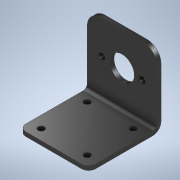
# Autodesk Inventor part: Pad dong co 775
Saved by Autodesk Inventor 2020 (Build 240168000, 168)
## iProperties
Created: 2021-05-25
Part Number: Pad dong co 775
Material: Generic
Document SubType Name: Sheet Metal
Designer: admin
Density: 1 g/cm^3
Sheet Metal Rule: Default_mm
Appearance: Glossy - Black
Author: admin
Autodesk Inventor part; units mm, degrees
ref_plane "YZ Plane" through (0, 0, 0) normal (1, 0, 0) x (0, 1, 0)
ref_plane "XZ Plane" through (0, 0, 0) normal (0, 1, 0) x (-1, 0, 0)
ref_plane "XY Plane" through (0, 0, 0) normal (0, 0, 1) x (1, 0, 0)
sketch "Sketch1" plane through (0, 0, 0) normal (0, 0, 1) x (1, 0, 0)
  line L0 (-25, -26) -> (25, -26)
  line L1 (25, -26) -> (25, 26)
  line L2 (25, 26) -> (-25, 26)
  line L3 (-25, 26) -> (-25, -26)
  line L4 (-25, -26) -> (25, 26) construction
  line L5 (25, -26) -> (-25, 26) construction
  circle A0 centre (0, 2) radius 8.8
  circle A1 centre (-14.5, 2) radius 2.25
  circle A2 centre (14.5, 2) radius 2.25
  point P0 (0, 0)
  dimension "d0" = 50
  dimension "d1" = 52
  dimension "d2" = 17.6
  dimension "d3" = 24
  dimension "d4" = 4.5
  dimension "d5" = 4.5
  dimension "d6" = 29
  dimension "d7" = 14.5
  dimension "d8" = 24
  dimension "d9" = 24
  dimension "d10" = 25
  measures "d0" distance of L2.end L1.end
  measures "d1" distance of L1.end L0.end
  measures "d2" diameter of A0
  measures "d3" distance from line of A0.centre L2
  measures "d4" diameter of A1
  measures "d5" diameter of A2
  measures "d6" distance of A2.centre A1.centre
  measures "d7" horizontal distance of A1.centre point (0, 0)
  measures "d8" distance from line of L2 A1.centre
  measures "d9" distance from line of L2 A2.centre
  measures "d10" distance from line of L3 A0.centre
extrude "Plate1" add sketch "Sketch1" along normal blind 3
sketch "Sketch2" plane through (25, -23, 0) normal (0, -1, 0) x (1, 0, 0)
  line L0 (-50, 0) -> (0, 0)
  line L1 (0, 0) -> (0, 52)
  line L2 (0, 52) -> (-50, 52)
  line L3 (-50, 52) -> (-50, 0)
  constraints: 6 end point, 1 horizontal, 1 perpendicular, 1 vertical
edge flange "Flange1" height 52 angle 90 thickness 3 bend radius 3 thickness toward (0, -1, 0) relief tear relief width 3 relief depth 1.5 edges at (0, -26, 3) wall of the first edge with corners at (-25, -23, 0) (25, -23, 0) (25, -23, 52) (-25, -23, 52)
bend "Bend1"
corner "Corner1"
fillet "Fillet1" radius 10 2 edges at (25, 26, 1.5) (-25, 26, 1.5)
fillet "Fillet2" radius 5 2 edges at (-25, -24.5, 52) (25, -24.5, 52)
sketch "Sketch3" plane through (-25, -26, 6) normal (0, -1, 0) x (1, 0, 0)
  line L0 (8.5, 38.5) -> (41.5, 38.5)
  line L1 (41.5, 38.5) -> (41.5, 5.5)
  line L2 (41.5, 5.5) -> (8.5, 5.5)
  line L3 (8.5, 5.5) -> (8.5, 38.5)
  line L4 (8.5, 38.5) -> (41.5, 5.5) construction
  line L5 (41.5, 38.5) -> (8.5, 5.5) construction
  line L6 (5, 46) -> (45, 46) projected
  line L7 (50, 41) -> (50, 0) projected
  circle A0 centre (41.5, 38.5) radius 2.25
  circle A1 centre (41.5, 5.5) radius 2.25
  circle A2 centre (8.5, 38.5) radius 2.25
  circle A3 centre (8.5, 5.5) radius 2.25
  point P0 (25, -6)
  point P1 (25, 22)
  dimension "d24" = 33
  dimension "d25" = 33
  dimension "d26" = 24
  dimension "d27" = 25
  dimension "d28" = 4.5
  dimension "d29" = 4.5
  dimension "d30" = 4.5
  dimension "d31" = 4.5
  constraints: 12 end point, 4 centre point, 4 coincident, 2 midpoint, 2 parallel, 1 horizontal, 1 perpendicular
  measures "d24" distance of L1.end L2.end
  measures "d25" distance of L0.end L1.end
  measures "d26" distance from line of L6 point (25, 22)
  measures "d27" distance from line of point (25, 22) L7
  measures "d28" diameter of A0
  measures "d29" diameter of A1
  measures "d30" diameter of A2
  measures "d31" diameter of A3
extrude "Cut1" cut sketch "Sketch3" against normal blind 3 contours L3 A2 L0 | L0 A2 L3 | A0 L1 L0 | L0 L1 A0 | A3 L2 L3 | L3 L2 A3 | A1 L2 L1 | L1 L2 A1
equation "\"d32\" = Thickness"
equation "\"d11\" = Thickness"
equation "\"d12\" = BendReliefWidth"
equation "\"d13\" = BendReliefDepth"
equation "\"d14\" = MinimumRemnant"
equation "\"d15\" = TransitionRadius"
equation "\"d18\" = BendRadius"
equation "\"d19\" = CornerReliefSize"
equation "\"d20\" = GapSize"
equation "\"d21\" = JacobiRadiusSize"
equation "\"BendRadius\" = Thickness"
equation "\"BendReliefWidth\" = Thickness"
equation "\"BendReliefDepth\" = 0.5 * Thickness"
equation "\"CornerReliefSize\" = 4 * Thickness"
equation "\"MinimumRemnant\" = 2 * Thickness"
equation "\"TransitionRadius\" = BendRadius"
equation "\"JacobiRadiusSize\" = BendRadius"
equation "\"GapSize\" = Thickness"
equation "\"Thickness\" = 3"
body "Solid1"
